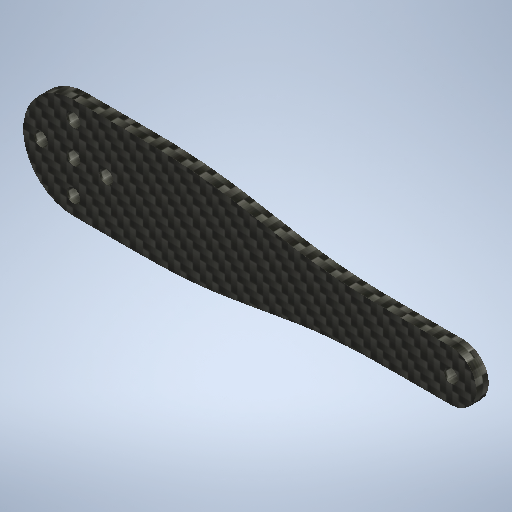
# Autodesk Inventor part: RT_ARM_MC_002
Saved by Autodesk Inventor 2025.4 (Build 294407000, 407)
## iProperties
Created: 2026-04-27
Part Number: RT_ARM_MC_002
Material: CFRP
Document SubType Name: Modeling
Designer: louis
Density: 1.43 g/cm^3
Appearance: Carbon Fiber 1
Author: louis
Autodesk Inventor part; units mm, degrees
ref_plane "YZ Plane" through (0, 0, 0) normal (1, 0, 0) x (0, 1, 0)
ref_plane "XZ Plane" through (0, 0, 0) normal (0, 1, 0) x (-1, 0, 0)
ref_plane "XY Plane" through (0, 0, 0) normal (0, 0, 1) x (1, 0, 0)
sketch "Sketch2" plane through (0, 0, 0) normal (0, 1, 0) x (-1, 0, 0)
  circle A0 centre (0, 0) radius 20
  circle A1 centre (-150, 0) radius 10
  line L0 (0, 0) -> (-150, 0)
  line L1 (0, 20) -> (-20, 20)
  line L2 (-150, 10) -> (-130, 10)
  spline S0 degree 4 poles (-20, 20) (-33.8351, 20) (-61.5052, 20) (-88.4948, 10) (-116.1649, 10) (-130, 10) knots 0 0 0 0 0 0.5 1 1 1 1 1
  line L3 (0, 0) -> (0, 20) construction
  line L4 (-150, 0) -> (-150, 10) construction
  line L5 (0, -20) -> (-20, -20)
  line L6 (-150, -10) -> (-130, -10)
  spline S1 degree 4 poles (-20, -20) (-33.8351, -20) (-61.5052, -20) (-88.4948, -10) (-116.1649, -10) (-130, -10) knots 0 0 0 0 0 0.5 1 1 1 1 1
  line L7 (13, 0) -> (-13, 0) construction
  point P0 (0, -20)
  point P1 (0, 13)
  point P2 (0, -13)
  dimension "d0" = 40
  dimension "d1" = 20
  dimension "d2" = 150
  dimension "d3" = 20
  dimension "d4" = 20
  dimension "d5" = 26
  dimension "d24" = 90
  constraints: 16 end point, 7 horizontal, 5 coincident, 4 symmetric about line, 2 vertical, 1 midpoint, 1 point on line, 13 other
  measures "d2" distance of L0.start L0.end
  measures "d3" distance of L1.start L1.end
  measures "d4" distance of L2.start L2.end
  measures "d5" distance of L7.start L7.end
extrude "Extrusion1" add sketch "Sketch2" along normal blind 5
hole "Hole1" at (-13, 0, 0) at (13, 0, 0) at (0, 0, 13) at (0, 0, -13) direction (0, 1, 0) diameter 5.5 end through all clearance for "Socket Head Cap Screw" size "M5" standard "Ansi Metric M Profile"
hole "Hole2" at (150, 0, 0) at (0, 0, 0) direction (0, 1, 0) diameter 5.5 end through all clearance for "Socket Head Cap Screw" size "M5" standard "Ansi Metric M Profile"
body "Solid1"
